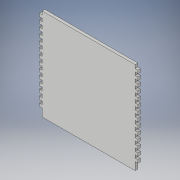
# Autodesk Inventor part: bottom-case
Saved by Autodesk Inventor 2019.4 (Build 234330000, 330)
## iProperties
Created: 2019-12-17
Part Number: bottom-case
Material: Generic
Document SubType Name: Modeling
Designer: fabfarm
Density: 1 g/cm^3
Appearance: Default
Author: fabfarm
Autodesk Inventor part; units mm, degrees
ref_plane "YZ Plane" through (0, 0, 0) normal (1, 0, 0) x (0, 1, 0)
ref_plane "XZ Plane" through (0, 0, 0) normal (0, 1, 0) x (-1, 0, 0)
ref_plane "XY Plane" through (0, 0, 0) normal (0, 0, 1) x (1, 0, 0)
sketch "Sketch1" plane through (0, 0, 0) normal (0, 0, 1) x (1, 0, 0)
  line L0 (330, -307.45) -> (-330, -307.45)
  line L1 (-330, -307.45) -> (-330, 307.45)
  line L2 (-330, 307.45) -> (330, 307.45)
  line L3 (330, 307.45) -> (330, -307.45)
  line L4 (330, -307.45) -> (-330, 307.45) construction
  line L5 (-330, -307.45) -> (330, 307.45) construction
  point P0 (0, 0)
  dimension "d0" = 614.9
  dimension "d1" = 660
  constraints: 12 end point, 2 midpoint, 2 parallel, 1 horizontal, 1 perpendicular
  measures "d0" distance of L2.end L0.start
  measures "d1" distance of L0.start L0.end
extrude "Extrusion1" add sketch "Sketch1" along normal blind 18.55
sketch "Sketch2" plane through (0, 0, 18.55) normal (0, 0, 1) x (1, 0, 0)
  line L0 (-330, 307.45) -> (-330, -307.45) projected
  line L1 (-330, 305) -> (-311.45, 305)
  line L2 (-311.45, 305) -> (-311.45, 285)
  line L3 (-311.45, 285) -> (-330, 285)
  line L4 (-330, 285) -> (-330, 305)
  line L5 (330, 307.45) -> (-330, 307.45) projected
  line L6 (-330, 265) -> (-311.45, 265)
  line L7 (-311.45, 265) -> (-311.45, 245)
  line L8 (-311.45, 245) -> (-330, 245)
  line L9 (-330, 245) -> (-330, 265)
  line L10 (-330, 225) -> (-311.45, 225)
  line L11 (-311.45, 225) -> (-311.45, 205)
  line L12 (-311.45, 205) -> (-330, 205)
  line L13 (-330, 205) -> (-330, 225)
  line L14 (-330, 185) -> (-311.45, 185)
  line L15 (-311.45, 185) -> (-311.45, 165)
  line L16 (-311.45, 165) -> (-330, 165)
  line L17 (-330, 165) -> (-330, 185)
  line L18 (-330, 145) -> (-311.45, 145)
  line L19 (-311.45, 145) -> (-311.45, 125)
  line L20 (-311.45, 125) -> (-330, 125)
  line L21 (-330, 125) -> (-330, 145)
  line L22 (-330, 105) -> (-311.45, 105)
  line L23 (-311.45, 105) -> (-311.45, 85)
  line L24 (-311.45, 85) -> (-330, 85)
  line L25 (-330, 85) -> (-330, 105)
  line L26 (-330, 65) -> (-311.45, 65)
  line L27 (-311.45, 65) -> (-311.45, 45)
  line L28 (-311.45, 45) -> (-330, 45)
  line L29 (-330, 45) -> (-330, 65)
  line L30 (-330, 25) -> (-311.45, 25)
  line L31 (-311.45, 25) -> (-311.45, 5)
  line L32 (-311.45, 5) -> (-330, 5)
  line L33 (-330, 5) -> (-330, 25)
  line L34 (-330, -15) -> (-311.45, -15)
  line L35 (-311.45, -15) -> (-311.45, -35)
  line L36 (-311.45, -35) -> (-330, -35)
  line L37 (-330, -35) -> (-330, -15)
  line L38 (-330, -55) -> (-311.45, -55)
  line L39 (-311.45, -55) -> (-311.45, -75)
  line L40 (-311.45, -75) -> (-330, -75)
  line L41 (-330, -75) -> (-330, -55)
  line L42 (-330, -95) -> (-311.45, -95)
  line L43 (-311.45, -95) -> (-311.45, -115)
  line L44 (-311.45, -115) -> (-330, -115)
  line L45 (-330, -115) -> (-330, -95)
  line L46 (-330, -135) -> (-311.45, -135)
  line L47 (-311.45, -135) -> (-311.45, -155)
  line L48 (-311.45, -155) -> (-330, -155)
  line L49 (-330, -155) -> (-330, -135)
  line L50 (-330, -175) -> (-311.45, -175)
  line L51 (-311.45, -175) -> (-311.45, -195)
  line L52 (-311.45, -195) -> (-330, -195)
  line L53 (-330, -195) -> (-330, -175)
  line L54 (-330, -215) -> (-311.45, -215)
  line L55 (-311.45, -215) -> (-311.45, -235)
  line L56 (-311.45, -235) -> (-330, -235)
  line L57 (-330, -235) -> (-330, -215)
  point P0 (0, 0)
  dimension "d4" = 2.45
  dimension "d5" = 20
  dimension "d6" = 18.55
  dimension "d9" = 40
  constraints: 112 end point, 2 parallel, 1 horizontal, 1 perpendicular, 1 point on line, 1 vertical, 104 other
  measures "d4" distance between parallel lines of L1 L5
  measures "d5" distance of L1.end L2.end
  measures "d6" distance of L2.end L3.end
  measures "d9" distance of L1.start L6.start
extrude "Extrusion2" cut sketch "Sketch2" against normal blind 18.55
mirror "Mirror1" about plane through (0, 0, 0) normal (1, 0, 0) of "Extrusion2"
sketch "Sketch3" plane through (0, 0, 18.55) normal (0, 0, 1) x (1, 0, 0)
  line L0 (-330, 305) -> (-330, 307.45) projected
  line L1 (-330, 305) -> (-311.45, 305) projected
  line L2 (-330, 307.45) -> (-311.45, 307.45)
  line L3 (-311.45, 307.45) -> (-311.45, 305)
  line L4 (-311.45, 305) -> (-330, 305)
  line L5 (-330, 305) -> (-330, 307.45)
  line L6 (311.45, 305) -> (330, 305) projected
  line L7 (-330, 307.45) -> (330, 307.45) projected
  line L8 (311.45, 305) -> (330, 305)
  line L9 (330, 305) -> (330, 307.45)
  line L10 (330, 307.45) -> (311.45, 307.45)
  line L11 (311.45, 307.45) -> (311.45, 305)
  point P0 (0, 0)
  constraints: 16 end point, 4 parallel, 2 horizontal, 2 perpendicular
extrude "Extrusion3" cut sketch "Sketch3" against normal blind 50
sketch "Sketch4" plane through (0, 0, 18.55) normal (0, 0, 1) x (1, 0, 0)
  line L0 (-330, -307.45) -> (330, -307.45) projected
  line L1 (-330, -307.45) -> (-311.45, -307.45)
  line L2 (-311.45, -307.45) -> (-311.45, -255)
  line L3 (-311.45, -255) -> (-330, -255)
  line L4 (-330, -255) -> (-330, -307.45)
  line L5 (-311.45, -215) -> (-311.45, -235) projected
  line L6 (-311.45, -235) -> (-330, -235) projected
  line L7 (330, -307.45) -> (311.45, -307.45)
  line L8 (311.45, -307.45) -> (311.45, -255)
  line L9 (311.45, -255) -> (330, -255)
  line L10 (330, -255) -> (330, -307.45)
  line L11 (311.45, -235) -> (311.45, -215) projected
  point P0 (0, 0)
  dimension "d18" = 20
  constraints: 16 end point, 4 parallel, 3 collinear, 2 horizontal, 2 perpendicular
  measures "d18" distance between parallel lines of L3 L6
extrude "Extrusion4" cut sketch "Sketch4" against normal blind 50
body "Solid1"
